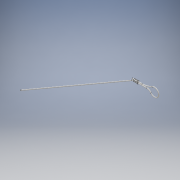
# Autodesk Inventor part: wire
Saved by Autodesk Inventor 2018 (Build 220112000, 112)
## iProperties
Created: 2018-06-15
Part Number: wire
Material: 一般
Document SubType Name: Modeling
Designer: KITformula
Density: 1 g/cm^3
Appearance: 既定
Author: KITformula
Autodesk Inventor part; units mm, degrees
ref_plane "YZ Plane" through (0, 0, 0) normal (1, 0, 0) x (0, 1, 0)
ref_plane "XZ Plane" through (0, 0, 0) normal (0, 1, 0) x (-1, 0, 0)
ref_plane "XY Plane" through (0, 0, 0) normal (0, 0, 1) x (1, 0, 0)
sketch "スケッチ1" plane through (0, 0, 0) normal (1, 0, 0) x (0, 1, 0)
  circle A0 centre (0, 0) radius 1.25
  dimension "d0" = 2.5
  constraints: 1 centre point, 1 coincident
  measures "d0" diameter of A0
extrude "押し出し1" add sketch "スケッチ1" along normal mid plane 30
sketch "スケッチ2" plane through (15, 0, 0) normal (1, 0, 0) x (0, 0, -1)
  circle A0 centre (0, 0) radius 1.25 projected
sketch "スケッチ3" plane through (0, 0, 0) normal (0, 1, 0) x (-1, 0, 0)
  line L0 (-15, 1.25) -> (-15, -1.25) projected
  arc A0 (-15, 0) -> (-25.7164, -5.7196) centre (-15, -12.8991) ccw
  arc A1 (-29.4041, 10.1723) -> (-25.7164, -5.7196) centre (-35, 0.5) ccw
  arc A2 (-29.4041, 10.1723) -> (-2.6845, 3) centre (-2.6845, 56.3563) ccw
  line L1 (-2.6845, 3) -> (7.3155, 3)
  point P0 (0, 0)
  dimension "d3" = 3
  dimension "d4" = 20
  dimension "d5" = 2.5
  dimension "d8" = 10
  constraints: 6 point on circle, 3 centre point, 3 tangent, 2 end point, 1 horizontal, 1 line through centre, 1 midpoint
  measures "d3" distance from line of A0.start L1
  measures "d4" distance from line of A1.centre L0
  measures "d5" distance from line of A1.centre L1
  measures "d8" distance of L1.start L1.end
sweep "スイープ1" add profiles "スケッチ2" path "スケッチ3" path curves A0 A1 A2 L1
sketch "スケッチ4" plane through (-7.3155, 0, 3) normal (-1, 0, 0) x (0, 0, 1)
  line L0 (-5, -2.5) -> (2, -2.5)
  line L1 (2, -2.5) -> (2, 2.5)
  line L2 (2, 2.5) -> (-5, 2.5)
  line L3 (-5, 2.5) -> (-5, -2.5)
  line L4 (-5, -2.5) -> (2, 2.5) construction
  line L5 (2, -2.5) -> (-5, 2.5) construction
  circle A0 centre (0, 0) radius 1.25 projected
  line L6 (-19.8942, 0) -> (14.8942, 0) projected
  point P0 (-3, 0)
  point P1 (-1.5, 0)
  point P2 (-1.5, 0)
  dimension "d9" = 1.5
  dimension "d10" = 7
  dimension "d11" = 5
  constraints: 12 end point, 3 midpoint, 2 parallel, 1 horizontal, 1 perpendicular, 1 point on line
  measures "d9" distance of A0.centre point (-1.5, 0)
  measures "d10" distance of L1.end L2.end
  measures "d11" distance of L2.end L0.start
extrude "押し出し2" add sketch "スケッチ4" along normal blind 10
fillet "フィレット1" radius 2 4 edges at (-12.3155, 2.5, -2) (-12.3155, -2.5, -2) (-12.3155, -2.5, 5) (-12.3155, 2.5, 5)
sketch "スケッチ5" plane through (-17.3155, 0, 3) normal (-1, 0, 0) x (0, 0, 1)
  circle A0 centre (0, 0) radius 1.25 projected
  point P0 (-3, 0)
extrude "押し出し3" add sketch "スケッチ5" along normal blind 5
sketch "スケッチ6" plane through (0, 0, 0) normal (0, 1, 0) x (-1, 0, 0)
  line L0 (15, -1.25) -> (15, 1.25) projected
  arc A0 (25, -2.6795) -> (15, 0) centre (15, -20) ccw
  line L1 (25, -2.6795) -> (314.5135, -169.8302)
  line L2 (7.3155, 1.25) -> (-15, 1.25) projected
  point P0 (0, 0)
  dimension "d17" = 30
  dimension "d18" = 20
  constraints: 2 end point, 2 point on circle, 1 centre point, 1 tangent, 3 other
  measures "d17" angle of L1 L2
  measures "d18" radius of A0
sketch "スケッチ7" plane through (-15, 0, 0) normal (-1, 0, 0) x (0, 0, 1)
  circle A0 centre (0, 0) radius 1.25 projected
sweep "スイープ2" add profiles "スケッチ7" path "スケッチ6" path curves A0 L1
